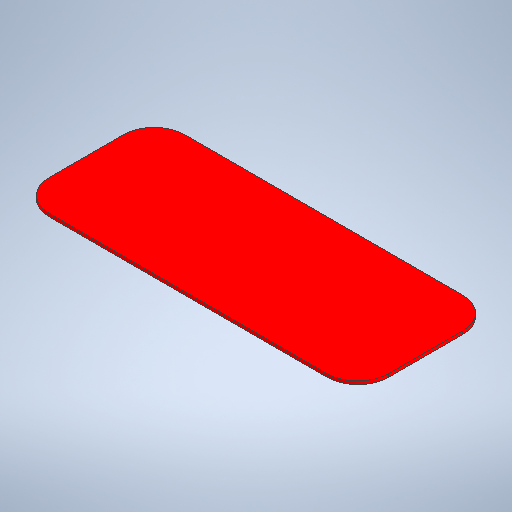
# Autodesk Inventor part: thermal pad
Saved by Autodesk Inventor 2025.2 (Build 292293000, 293)
## iProperties
Created: 2024-11-29
Part Number: thermal pad
Material: Generic
Document SubType Name: Modeling
Designer: cbast
Density: 1 g/cm^3
Appearance: Default
Author: cbast
Autodesk Inventor part; units mm, degrees
ref_plane "YZ Plane" through (0, 0, 0) normal (1, 0, 0) x (0, 1, 0)
ref_plane "XZ Plane" through (0, 0, 0) normal (0, 1, 0) x (-1, 0, 0)
ref_plane "XY Plane" through (0, 0, 0) normal (0, 0, 1) x (1, 0, 0)
sketch "Sketch1" plane through (0, 0, 0) normal (0, 1, 0) x (-1, 0, 0)
  line L0 (45, 22) -> (-45, 22)
  line L1 (-55, 12) -> (-55, -12)
  line L2 (-45, -22) -> (45, -22)
  line L3 (55, -12) -> (55, 12)
  line L4 (55, 22) -> (-55, -22) construction
  line L5 (-55, 22) -> (55, -22) construction
  arc A0 (55, 12) -> (45, 22) centre (45, 12) ccw
  arc A1 (45, -22) -> (55, -12) centre (45, -12) ccw
  arc A2 (-55, -12) -> (-45, -22) centre (-45, -12) ccw
  arc A3 (-45, 22) -> (-55, 12) centre (-45, 12) ccw
  point P0 (0, 0)
  dimension "d0" = 110
  dimension "d1" = 44
  dimension "d2" = 10
  dimension "d3" = 10
  dimension "d4" = 10
  constraints: 12 end point, 8 point on circle, 8 point on line, 8 tangent, 4 centre point, 2 midpoint, 2 parallel, 1 equal radius, 1 horizontal, 1 perpendicular
  measures "d0" distance of L5.end L4.end
  measures "d1" distance of L4.end L5.start
  measures "d2" radius of A0
  measures "d3" radius of A1
  measures "d4" radius of A2
extrude "Extrusion1" add sketch "Sketch1" along normal blind 1
body "Solid1"
